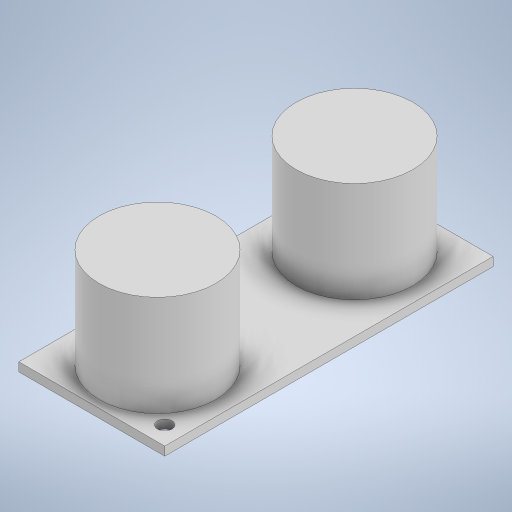
# Autodesk Inventor part: 초음파센서
Saved by Autodesk Inventor 2024 (Build 280153000, 153)
## iProperties
Created: 2024-04-20
Part Number: 초음파센서
Material: 일반
Document SubType Name: Modeling
Designer: ckhye
Density: 1 g/cm^3
Appearance: 기본값
Author: ckhye
Autodesk Inventor part; units mm, degrees
ref_plane "YZ Plane" through (0, 0, 0) normal (1, 0, 0) x (0, 1, 0)
ref_plane "XZ Plane" through (0, 0, 0) normal (0, 1, 0) x (-1, 0, 0)
ref_plane "XY Plane" through (0, 0, 0) normal (0, 0, 1) x (1, 0, 0)
sketch "스케치1" plane through (0, 0, 0) normal (0, 1, 0) x (-1, 0, 0)
  line L0 (10, 22.5) -> (-10, 22.5)
  line L1 (-10, 22.5) -> (-10, -22.5)
  line L2 (-10, -22.5) -> (10, -22.5)
  line L3 (10, -22.5) -> (10, 22.5)
  line L4 (10, 22.5) -> (-10, -22.5) construction
  line L5 (-10, 22.5) -> (10, -22.5) construction
  line L6 (-7.5, 20) -> (-7.5, -20) construction
  line L7 (0, 13.5) -> (0, -13.5) construction
  circle A0 centre (0, 13.5) radius 8
  circle A1 centre (0, -13.5) radius 8
  line L8 (7.5, 20) -> (7.5, -20) construction
  circle A2 centre (-7.5, 20) radius 1
  circle A3 centre (7.5, -20) radius 1
  point P0 (0, 0)
  point P1 (0, 0)
  dimension "d0" = 20
  dimension "d1" = 45
  dimension "d2" = 27
  dimension "d3" = 40
  dimension "d4" = 20
  dimension "d5" = 10
  dimension "d6" = 9
  dimension "d7" = 16
  dimension "d8" = 16
  dimension "d9" = 40
  dimension "d10" = 20
  dimension "d11" = 15
  dimension "d12" = 7.5
  dimension "d13" = 2
  dimension "d14" = 2
  constraints: 18 end point, 4 centre point, 4 coincident, 3 midpoint, 3 vertical, 2 parallel, 1 horizontal, 1 perpendicular
  measures "d0" distance of L2.end L1.end
  measures "d1" distance between parallel lines of L2 L0
  measures "d2" distance of L7.end L7.start
  measures "d3" distance of L6.end L6.start
  measures "d4" vertical distance of point (0, 0) L6.start
  measures "d5" distance from line of L3 L7.start
  measures "d6" distance from line of L0 L7.start
  measures "d7" diameter of A0
  measures "d8" diameter of A1
  measures "d9" distance of L8.end L8.start
  measures "d10" vertical distance of point (0, 0) L8.start
  measures "d11" distance between parallel lines of L6 L8
  measures "d12" distance from line of point (0, 0) L8
  measures "d13" diameter of A2
  measures "d14" diameter of A3
extrude "돌출1" add sketch "스케치1" along normal blind 1.2 contours L3 L2 L1 L0 | A0 | A1
sketch "스케치2" plane through (0, 1.2, 0) normal (0, 1, 0) x (1, 0, 0)
  line L0 (0, -13.5) -> (0, 13.5)
  line L1 (-10, 22.5) -> (-10, -22.5) projected
  line L2 (10, -22.5) -> (10, 22.5) projected
  circle A0 centre (0, -13.5) radius 8
  circle A1 centre (0, 13.5) radius 8
  point P0 (0, 0)
  point P1 (-10, 0)
  dimension "d17" = 27
  dimension "d20" = 10
  dimension "d21" = 13.5
  dimension "d22" = 16
  dimension "d23" = 16
  constraints: 2 centre point, 2 coincident, 2 end point, 1 midpoint, 1 vertical
  measures "d17" distance of L0.start L0.end
  measures "d20" distance from line of L2 L0.start
  measures "d21" distance of point (0, 0) L0.start
  measures "d22" diameter of A0
  measures "d23" diameter of A1
extrude "돌출2" add sketch "스케치2" along normal blind 13.8
